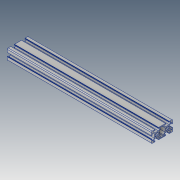
# Autodesk Inventor part: 200-40-BOGIE-CONNECTOR-P-01
Saved by Autodesk Inventor 2018.2 (Build 222227000, 227)
## iProperties
Manager: feesmrt
Company: FRANC0R
Created: 2017-11-20
Part Number: 200-40-BOGIE-CONNECTOR-P-01
Material: Aluminium 6061
Document SubType Name: Modeling
Designer: feesmrt
Density: 2.7 g/cm^3
Appearance: Aluminium - flach
Project: Rescue Robot
Cost Center: -
Description: Bogie Wheel Distance Profile
Engineer: feesmrt
Authority: feesmrt
Stock Number: 200-40-BOGIE-CONNECTOR-P-01
Author: feesmrt
Title: Bogie Wheel Distance Profile
Subject: Rescue Robot
Revision Number: 1
Autodesk Inventor part; units mm, degrees
ref_plane "YZ Plane" through (0, 0, 0) normal (1, 0, 0) x (0, 1, 0)
ref_plane "XZ Plane" through (0, 0, 0) normal (0, 1, 0) x (-1, 0, 0)
ref_plane "XY Plane" through (0, 0, 0) normal (0, 0, 1) x (1, 0, 0)
derived "90-50-PROFILES-20x40xSketch.ipt"
sketch "Skizze2" plane through (0, 0, 0) normal (1, 0, 0) x (0, 1, 0)
  line L0 (-6.5607, 4.5) -> (-4, 7.0607)
  line L1 (-13.4393, 4.5) -> (-6.5607, 4.5)
  line L2 (-16, 7.0607) -> (-13.4393, 4.5)
  line L3 (-16, 8.5) -> (-16, 7.0607)
  line L4 (-13, 8.5) -> (-16, 8.5)
  line L5 (-13, 9.5) -> (-13, 8.5)
  line L6 (-13.5, 9.5) -> (-13, 9.5)
  line L7 (-13.5, 10) -> (-13.5, 9.5)
  line L8 (-18.5, 10) -> (-13.5, 10)
  arc A0 (-18.5, 10) -> (-20, 8.5) centre (-18.5, 8.5) ccw
  line L9 (-20, 3.5) -> (-20, 8.5)
  line L10 (-19.5, 3.5) -> (-20, 3.5)
  line L11 (-19.5, 3) -> (-19.5, 3.5)
  line L12 (-18.5, 3) -> (-19.5, 3)
  line L13 (-18.5, 6) -> (-18.5, 3)
  line L14 (-17.0607, 6) -> (-18.5, 6)
  line L15 (-14.5, 3.4393) -> (-17.0607, 6)
  line L16 (-14.5, -3.4393) -> (-14.5, 3.4393)
  line L17 (-17.0607, -6) -> (-14.5, -3.4393)
  line L18 (-18.5, -6) -> (-17.0607, -6)
  line L19 (-18.5, -3) -> (-18.5, -6)
  line L20 (-19.5, -3) -> (-18.5, -3)
  line L21 (-19.5, -3.5) -> (-19.5, -3)
  line L22 (-20, -3.5) -> (-19.5, -3.5)
  line L23 (-20, -8.5) -> (-20, -3.5)
  arc A1 (-20, -8.5) -> (-18.5, -10) centre (-18.5, -8.5) ccw
  line L24 (-13.5, -10) -> (-18.5, -10)
  line L25 (-13.5, -9.5) -> (-13.5, -10)
  line L26 (-13, -9.5) -> (-13.5, -9.5)
  line L27 (-13, -8.5) -> (-13, -9.5)
  line L28 (-16, -8.5) -> (-13, -8.5)
  line L29 (-16, -7.0607) -> (-16, -8.5)
  line L30 (-13.4393, -4.5) -> (-16, -7.0607)
  line L31 (-6.5607, -4.5) -> (-13.4393, -4.5)
  line L32 (-4, -7.0607) -> (-6.5607, -4.5)
  line L33 (-4, -8.5) -> (-4, -7.0607)
  line L34 (-7, -8.5) -> (-4, -8.5)
  line L35 (-7, -9.5) -> (-7, -8.5)
  line L36 (-6.5, -9.5) -> (-7, -9.5)
  line L37 (-6.5, -10) -> (-6.5, -9.5)
  line L38 (6.5, -10) -> (-6.5, -10)
  line L39 (6.5, -9.5) -> (6.5, -10)
  line L40 (7, -9.5) -> (6.5, -9.5)
  line L41 (7, -8.5) -> (7, -9.5)
  line L42 (4, -8.5) -> (7, -8.5)
  line L43 (4, -7.0607) -> (4, -8.5)
  line L44 (6.5607, -4.5) -> (4, -7.0607)
  line L45 (13.4393, -4.5) -> (6.5607, -4.5)
  line L46 (16, -7.0607) -> (13.4393, -4.5)
  line L47 (16, -8.5) -> (16, -7.0607)
  line L48 (13, -8.5) -> (16, -8.5)
  line L49 (13, -9.5) -> (13, -8.5)
  line L50 (13.5, -9.5) -> (13, -9.5)
  line L51 (13.5, -10) -> (13.5, -9.5)
  line L52 (18.5, -10) -> (13.5, -10)
  arc A2 (18.5, -10) -> (20, -8.5) centre (18.5, -8.5) ccw
  line L53 (20, -3.5) -> (20, -8.5)
  line L54 (19.5, -3.5) -> (20, -3.5)
  line L55 (19.5, -3) -> (19.5, -3.5)
  line L56 (18.5, -3) -> (19.5, -3)
  line L57 (18.5, -6) -> (18.5, -3)
  line L58 (17.0607, -6) -> (18.5, -6)
  line L59 (14.5, -3.4393) -> (17.0607, -6)
  line L60 (14.5, 3.4393) -> (14.5, -3.4393)
  line L61 (17.0607, 6) -> (14.5, 3.4393)
  line L62 (18.5, 6) -> (17.0607, 6)
  line L63 (18.5, 3) -> (18.5, 6)
  line L64 (19.5, 3) -> (18.5, 3)
  line L65 (19.5, 3.5) -> (19.5, 3)
  line L66 (20, 3.5) -> (19.5, 3.5)
  line L67 (20, 8.5) -> (20, 3.5)
  arc A3 (20, 8.5) -> (18.5, 10) centre (18.5, 8.5) ccw
  line L68 (13.5, 10) -> (18.5, 10)
  line L69 (13.5, 9.5) -> (13.5, 10)
  line L70 (13, 9.5) -> (13.5, 9.5)
  line L71 (13, 8.5) -> (13, 9.5)
  line L72 (16, 8.5) -> (13, 8.5)
  line L73 (16, 7.0607) -> (16, 8.5)
  line L74 (13.4393, 4.5) -> (16, 7.0607)
  line L75 (6.5607, 4.5) -> (13.4393, 4.5)
  line L76 (4, 7.0607) -> (6.5607, 4.5)
  line L77 (4, 8.5) -> (4, 7.0607)
  line L78 (7, 8.5) -> (4, 8.5)
  line L79 (7, 9.5) -> (7, 8.5)
  line L80 (6.5, 9.5) -> (7, 9.5)
  line L81 (6.5, 10) -> (6.5, 9.5)
  line L82 (-6.5, 10) -> (6.5, 10)
  line L83 (-6.5, 9.5) -> (-6.5, 10)
  line L84 (-7, 9.5) -> (-6.5, 9.5)
  line L85 (-7, 8.5) -> (-7, 9.5)
  line L86 (-4, 8.5) -> (-7, 8.5)
  line L87 (-4, 7.0607) -> (-4, 8.5)
  line L88 (-2.5, 6.4393) -> (-2.5, 8.5)
  line L89 (-2.5, 8.5) -> (2.5, 8.5)
  line L90 (2.5, 8.5) -> (2.5, 6.4393)
  line L91 (2.5, 6.4393) -> (5.5, 3.4393)
  line L92 (5.5, 3.4393) -> (5.5, -3.4393)
  line L93 (5.5, -3.4393) -> (2.5, -6.4393)
  line L94 (2.5, -6.4393) -> (2.5, -8.5)
  line L95 (2.5, -8.5) -> (-2.5, -8.5)
  line L96 (-2.5, -8.5) -> (-2.5, -6.4393)
  line L97 (-2.5, -6.4393) -> (-5.5, -3.4393)
  line L98 (-5.5, -3.4393) -> (-5.5, 3.4393)
  line L99 (-5.5, 3.4393) -> (-2.5, 6.4393)
  arc A4 (11.2768, 2.4356) -> (8.7232, 2.4356) centre (10, 0) ccw
  line L100 (11.2768, 2.4356) -> (11.9496, 3.0002)
  line L101 (11.9496, 3.0002) -> (13.0002, 1.9496)
  line L102 (13.0002, 1.9496) -> (12.4356, 1.2768)
  arc A5 (12.4356, -1.2768) -> (12.4356, 1.2768) centre (10, 0) ccw
  line L103 (12.4356, -1.2768) -> (13.0002, -1.9496)
  line L104 (13.0002, -1.9496) -> (11.9496, -3.0002)
  line L105 (11.9496, -3.0002) -> (11.2768, -2.4356)
  arc A6 (8.7232, -2.4356) -> (11.2768, -2.4356) centre (10, 0) ccw
  line L106 (8.7232, -2.4356) -> (8.0504, -3.0002)
  line L107 (8.0504, -3.0002) -> (6.9998, -1.9496)
  line L108 (6.9998, -1.9496) -> (7.5644, -1.2768)
  arc A7 (7.5644, 1.2768) -> (7.5644, -1.2768) centre (10, 0) ccw
  line L109 (7.5644, 1.2768) -> (6.9998, 1.9496)
  line L110 (6.9998, 1.9496) -> (8.0504, 3.0002)
  line L111 (8.0504, 3.0002) -> (8.7232, 2.4356)
  arc A8 (-8.7232, 2.4356) -> (-11.2768, 2.4356) centre (-10, 0) ccw
  line L112 (-8.7232, 2.4356) -> (-8.0504, 3.0002)
  line L113 (-8.0504, 3.0002) -> (-6.9998, 1.9496)
  line L114 (-6.9998, 1.9496) -> (-7.5644, 1.2768)
  arc A9 (-7.5644, -1.2768) -> (-7.5644, 1.2768) centre (-10, 0) ccw
  line L115 (-7.5644, -1.2768) -> (-6.9998, -1.9496)
  line L116 (-6.9998, -1.9496) -> (-8.0504, -3.0002)
  line L117 (-8.0504, -3.0002) -> (-8.7232, -2.4356)
  arc A10 (-11.2768, -2.4356) -> (-8.7232, -2.4356) centre (-10, 0) ccw
  line L118 (-11.2768, -2.4356) -> (-11.9496, -3.0002)
  line L119 (-11.9496, -3.0002) -> (-13.0002, -1.9496)
  line L120 (-13.0002, -1.9496) -> (-12.4356, -1.2768)
  arc A11 (-12.4356, 1.2768) -> (-12.4356, -1.2768) centre (-10, 0) ccw
  line L121 (-12.4356, 1.2768) -> (-13.0002, 1.9496)
  line L122 (-13.0002, 1.9496) -> (-11.9496, 3.0002)
  line L123 (-11.9496, 3.0002) -> (-11.2768, 2.4356)
  point P0 (0, 0)
extrude "Extrusion4" add sketch "Skizze2" along normal mid plane 270
